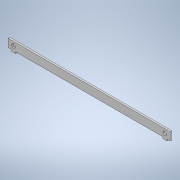
# Autodesk Inventor part: 零件1
Saved by Autodesk Inventor 2022.3 (Build 263350000, 350)
## iProperties
Created: 2023-04-16
Part Number: 零件1
Material: 一般
Document SubType Name: Modeling
Designer: JOU
Density: 1 g/cm^3
Appearance: 預設
Author: JOU
Autodesk Inventor part; units mm, degrees
ref_plane "YZ Plane" through (0, 0, 0) normal (1, 0, 0) x (0, 1, 0)
ref_plane "XZ Plane" through (0, 0, 0) normal (0, 1, 0) x (-1, 0, 0)
ref_plane "XY Plane" through (0, 0, 0) normal (0, 0, 1) x (1, 0, 0)
sketch "草圖1" plane through (0, 0, 0) normal (0, 0, 1) x (1, 0, 0)
  line L0 (0, 15) -> (300, 15)
  line L1 (300, 15) -> (300, 0)
  line L2 (300, 0) -> (0, 0)
  line L3 (0, 0) -> (0, 15)
  circle A0 centre (10, 7.5) radius 3.5
  circle A1 centre (290, 7.5) radius 3.5
  line L4 (6, 0) -> (14, 0)
  line L5 (14, 0) -> (14, -2.9)
  line L6 (14, -2.9) -> (6, -2.9)
  line L7 (6, -2.9) -> (6, 0)
  line L8 (286, 0) -> (294, 0)
  line L9 (294, 0) -> (294, -2.9)
  line L10 (294, -2.9) -> (286, -2.9)
  line L11 (286, -2.9) -> (286, 0)
  point P0 (6, -1.45)
  point P1 (294, -1.45)
  point P2 (294, 0)
  dimension "d0" = 300
  dimension "d1" = 15
  dimension "d2" = 7.5
  dimension "d3" = 7
  dimension "d4" = 10
  dimension "d5" = 10
  dimension "d6" = 7.5
  dimension "d7" = 7
  dimension "d10" = 6
  dimension "d11" = 6
  dimension "d12" = 8
  dimension "d13" = 2.9
  dimension "d14" = 8
  constraints: 24 end point, 6 parallel, 3 horizontal, 3 perpendicular, 3 point on line, 2 centre point, 2 midpoint, 1 coincident
  measures "d0" distance of L0.start L0.end
  measures "d1" distance of L2.end L0.start
  measures "d2" distance from line of L0 A0.centre
  measures "d3" diameter of A0
  measures "d4" distance from line of L3 A0.centre
  measures "d5" distance from line of A1.centre L1
  measures "d6" distance from line of L0 A1.centre
  measures "d7" diameter of A1
  measures "d10" distance from line of point (6, -1.45) L3
  measures "d11" distance from line of L1 point (294, -1.45)
  measures "d12" distance of L5.end L6.end
  measures "d13" distance of L4.end L5.end
  measures "d14" distance of L9.end L10.end
extrude "擠出1" add sketch "草圖1" along normal blind 3
